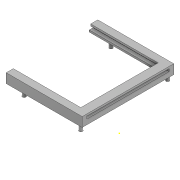
# Autodesk Inventor part: podstawa_2
Saved by Autodesk Inventor 2021 (Build 250183000, 183)
## iProperties
Created: 2022-06-23
Part Number: podstawa_2
Material: Generic
Document SubType Name: Modeling
Designer: agnpi
Density: 1 g/cm^3
Appearance: Orange
Author: agnpi
Autodesk Inventor part; units mm, degrees
ref_plane "YZ Plane" through (0, 0, 0) normal (1, 0, 0) x (0, 1, 0)
ref_plane "XZ Plane" through (0, 0, 0) normal (0, 1, 0) x (-1, 0, 0)
ref_plane "XY Plane" through (0, 0, 0) normal (0, 0, 1) x (1, 0, 0)
sketch "Sketch1" plane through (0, 0, 0) normal (0, 1, 0) x (-1, 0, 0)
  line L0 (164.8, 0) -> (-148.8, 0) projected
  line L1 (0, -144.2) -> (0, 144.2) projected
  line L2 (-80, 95) -> (80, 95)
  line L3 (80, 95) -> (80, -95)
  line L4 (80, -95) -> (-80, -95)
  line L5 (-80, -95) -> (-80, 95)
  line L6 (-80, 95) -> (80, -95) construction
  line L7 (80, 95) -> (-80, -95) construction
  line L8 (-88, 103) -> (88, 103)
  line L9 (88, 103) -> (88, -103)
  line L10 (88, -103) -> (-88, -103)
  line L11 (-88, -103) -> (-88, 103)
  point P0 (0, 0)
  dimension "d0" = 160
  dimension "d1" = 190
  dimension "d2" = 8
  dimension "d3" = 8
  dimension "d4" = 8
  dimension "d5" = 8
  constraints: 20 end point, 3 parallel, 3 perpendicular, 2 horizontal, 2 midpoint
  measures "d0" distance of L3.end L4.end
  measures "d1" distance of L2.end L3.end
  measures "d2" distance between parallel lines of L2 L8
  measures "d3" distance between parallel lines of L10 L4
  measures "d4" distance between parallel lines of L11 L5
  measures "d5" distance between parallel lines of L9 L3
extrude "Extrusion1" add sketch "Sketch1" along normal blind 8 contours L3 L4 L1 L0 | L0 L1 L2 L3 | L1 L4 L5 L0 | L0 L5 L2 L1
extrude "Extrusion2" add sketch "Sketch1" along normal blind 80 contours L9 L10 L1 L4 L3 L0 | L0 L3 L2 L1 L8 L9 | L1 L2 L5 L0 L11 L8 | L10 L11 L0 L5 L4 L1
move faces "Move1" translate (-16, 0, 0) faces at (80, 32, -31.6667)
move faces "Move5" translate (-8, 0, 0) faces at (88, 53.3333, 34.3333)
move faces "Move6" translate (-8, 0, 0) faces at (80, 53.3333, 34.3333)
move faces "Move7" translate (0, 0, -8) faces at (-32, 56, 95)
move faces "Move8" translate (0, 0, -8) faces at (-34.6667, 26.6667, 103)
move faces "Move9" translate (0, 0, -8) faces at (-32, 56, 87)
move faces "Move10" translate (0, 0, -8) faces at (-34.6667, 26.6667, 95)
thicken "Thicken1" operation add thickness 3 both sides no extend neighbours yes toward (0, 0, 1) faces at (-34.6667, 26.6667, 87)
thicken "Thicken3" operation add thickness 3 both sides no extend neighbours yes toward (0, 0, -1) faces at (18.6667, 26.6667, -103)
sketch "Sketch5" plane through (0, 8, 0) normal (0, 1, 0) x (1, 0, 0)
  line L0 (-80, -79) -> (-80, 95) projected
  line L1 (-80, 95) -> (64, 95) projected
  line L2 (-80, 89.3431) -> (-74.3431, 95)
  line L3 (-80, 89.3431) -> (-80, 95)
  line L4 (58.3431, 95) -> (64, 89.3431)
  line L5 (64, 95) -> (64, -79) projected
  line L6 (-80, -73.3431) -> (-74.3431, -79)
  line L7 (64, -79) -> (-80, -79) projected
  line L8 (58.3431, -79) -> (64, -73.3431)
  point P0 (0, 0)
  dimension "d69" = 45
  dimension "d70" = 8
  dimension "d73" = 8
  dimension "d74" = 45
  dimension "d75" = 8
  dimension "d76" = 45
  dimension "d77" = 8
  dimension "d78" = 45
  constraints: 10 end point, 8 point on line, 1 collinear
  measures "d69" angle of L2 L0
  measures "d70" distance of L2.start L2.end
  measures "d73" distance of L4.start L4.end
  measures "d74" angle of L5 L4
  measures "d75" distance of L6.start L6.end
  measures "d76" angle of L7 L6
  measures "d77" distance of L8.start L8.end
  measures "d78" angle of L7 L8
thicken "Thicken4" operation add thickness 1 both sides no extend neighbours yes toward (1, 0, 0) faces at (-80, 56, -37)
thicken "Thicken5" operation add thickness 1 both sides no extend neighbours yes toward (-1, 0, 0) faces at (64, 56, 21)
sketch "Sketch6" plane through (0, 0, 0) normal (0, -1, 0) x (1, 0, 0)
  line L0 (72, 90) -> (72, -106) projected
  line L1 (72, -106) -> (-88, -106) projected
  line L2 (72, 90) -> (-88, 90)
  line L3 (-88, 90) -> (-88, -106)
  line L4 (-88, -106) -> (72, -106)
  line L5 (72, -106) -> (72, 90)
  point P0 (0, 0)
  constraints: 8 end point, 2 parallel, 1 horizontal, 1 perpendicular
extrude "Extrusion7" cut sketch "Sketch6" against normal blind 45
sketch "Sketch7" plane through (-79, 80, 79) normal (1, 0, 0) x (0, 0, -1)
  line L0 (0, -35) -> (0, 0) projected
  line L1 (174, -13.5) -> (174, -21.5)
  line L2 (174, -21.5) -> (0, -21.5)
  line L3 (0, -21.5) -> (0, -13.5)
  line L4 (174, -35) -> (174, 0) projected
  line L5 (0, 0) -> (174, 0) projected
  line L6 (0, -13.5) -> (174, -13.5)
  point P0 (79, -80)
  point P1 (174, -17.5)
  point P2 (0, -21.5)
  dimension "d91" = 8
  constraints: 8 end point, 2 midpoint, 2 point on line, 1 horizontal, 1 parallel
  measures "d91" distance between parallel lines of L2 L6
extrude "Extrusion8" add sketch "Sketch7" along normal up to surface (142 mm away) contours L0 L6 L1 L2
sketch "Sketch8" plane through (-79, 66.5, 79) normal (0, 1, 0) x (1, 0, 0)
  line L0 (8, 166) -> (134, 166)
  line L1 (134, 166) -> (134, 8)
  line L2 (134, 8) -> (8, 8)
  line L3 (8, 8) -> (8, 166)
  line L4 (0, 174) -> (142, 174) projected
  line L5 (0, 0) -> (0, 174) projected
  line L6 (142, 0) -> (0, 0) projected
  line L7 (142, 174) -> (142, 0) projected
  point P0 (79, 79)
  dimension "d95" = 8
  dimension "d96" = 8
  dimension "d97" = 8
  dimension "d98" = 8
  constraints: 8 end point, 2 parallel, 1 horizontal, 1 perpendicular
  measures "d95" distance between parallel lines of L4 L0
  measures "d96" distance between parallel lines of L3 L5
  measures "d97" distance between parallel lines of L6 L2
  measures "d98" distance between parallel lines of L1 L7
extrude "Extrusion9" cut sketch "Sketch8" against normal through all contours L0 L1 L2 L3
sketch "Sketch10" plane through (-79, 80, 79) normal (1, 0, 0) x (0, 0, -1)
  line L0 (0, 0) -> (174, 0) projected
  line L1 (0, 0) -> (174, 0)
  line L2 (174, 0) -> (174, -4)
  line L3 (174, -4) -> (0, -4)
  line L4 (0, -4) -> (0, 0)
  line L5 (174, -13.5) -> (174, 0) projected
  point P0 (79, -80)
  point P1 (174, -6.75)
  dimension "d101" = 4
  constraints: 8 end point, 2 parallel, 1 horizontal, 1 midpoint, 1 perpendicular, 1 point on line
  measures "d101" distance between parallel lines of L0 L3
extrude "Extrusion10" add sketch "Sketch10" along normal up to surface (142 mm away)
sketch "Sketch11" plane through (0, 80, 0) normal (0, 1, 0) x (1, 0, 0)
  line L0 (53, 90) -> (-69, 90)
  line L1 (-69, 90) -> (-69, -74)
  line L2 (-69, -74) -> (53, -74)
  line L3 (53, -74) -> (53, 90)
  line L4 (72, -90) -> (72, 106) projected
  line L5 (72, 106) -> (-88, 106) projected
  line L6 (-88, -90) -> (72, -90) projected
  line L7 (-88, 106) -> (-88, -90) projected
  point P0 (0, 0)
  dimension "d104" = 19
  dimension "d105" = 16
  dimension "d106" = 16
  dimension "d107" = 19
  constraints: 8 end point, 2 parallel, 1 horizontal, 1 perpendicular
  measures "d104" distance between parallel lines of L4 L3
  measures "d105" distance between parallel lines of L5 L0
  measures "d106" distance between parallel lines of L6 L2
  measures "d107" distance between parallel lines of L7 L1
extrude "Extrusion11" cut sketch "Sketch11" against normal blind 8 contours L3 L2 L1 L0
sketch "Sketch12" plane through (63, 66.5, -95) normal (-1, 0, 0) x (0, 0, 1)
  line L0 (0, 0) -> (0, 9.5) projected
  line L1 (0, 0) -> (174, 0) projected
  line L2 (0, 9.5) -> (174, 9.5)
  line L3 (174, 9.5) -> (174, 0)
  line L4 (174, 0) -> (0, 0)
  line L5 (0, 0) -> (0, 9.5)
  point P0 (95, -66.5)
  constraints: 8 end point, 2 parallel, 1 horizontal, 1 perpendicular
extrude "Extrusion12" cut sketch "Sketch12" against normal through all
sketch "Sketch13" plane through (0, 80, 0) normal (0, 1, 0) x (1, 0, 0)
  line L0 (-69, 90) -> (-69, -74) projected
  line L1 (-69, -74) -> (-88, -74)
  line L2 (-69, 90) -> (-88, 90)
  line L3 (-88, -74) -> (-88, 90)
  line L4 (-88, 106) -> (-88, -90) projected
  line L5 (-69, 90) -> (-69, -74)
  point P0 (0, 0)
  constraints: 8 end point, 3 collinear, 2 horizontal
extrude "Extrusion13" cut sketch "Sketch13" against normal through all
sketch "Sketch14" plane through (-88, 80, -90) normal (0, 0, 1) x (1, 0, 0)
  line L0 (9, -13.5) -> (19, -13.5) projected
  line L1 (0, -35) -> (0, 0) projected
  line L2 (9, -13.5) -> (0, -13.5)
  line L3 (0, -13.5) -> (0, -4)
  line L4 (0, -4) -> (9, -4)
  line L5 (9, -4) -> (9, -13.5)
  point P0 (88, -80)
  constraints: 8 end point, 2 parallel, 2 point on line, 1 horizontal, 1 perpendicular
extrude "Extrusion14" cut sketch "Sketch14" against normal up to surface (5 mm away)
sketch "Sketch15" plane through (-69, 58.5, -90) normal (-1, 0, 0) x (0, 0, 1)
  line L0 (0, 8) -> (0, 0) projected
  line L1 (161, 0) -> (3, 0) projected
  line L2 (0, 8) -> (3, 8)
  line L3 (3, 8) -> (3, 0)
  line L4 (3, 0) -> (0, 0)
  line L5 (0, 0) -> (0, 8)
  point P0 (90, -58.5)
  constraints: 8 end point, 2 parallel, 1 horizontal, 1 perpendicular
extrude "Extrusion15" add sketch "Sketch15" along normal up to surface (19 mm away)
sketch "Sketch16" plane through (-69, 58.5, 71) normal (-1, 0, 0) x (0, 0, 1)
  line L0 (0, 8) -> (3, 8)
  line L1 (3, 8) -> (3, 0)
  line L2 (3, 0) -> (0, 0)
  line L3 (0, 0) -> (0, 8)
  point P0 (-71, -58.5)
  constraints: 8 end point, 2 parallel, 1 horizontal, 1 perpendicular
extrude "Extrusion16" add sketch "Sketch16" along normal up to surface (19 mm away)
sketch "Sketch17" plane through (53, 80, 74) normal (0, 0, -1) x (-1, 0, 0)
  line L0 (132, -13.5) -> (132, -4) projected
  line L1 (132, -13.5) -> (141, -13.5) projected
  line L2 (132, -4) -> (141, -4)
  line L3 (141, -4) -> (141, -13.5)
  line L4 (141, -13.5) -> (132, -13.5)
  line L5 (132, -13.5) -> (132, -4)
  line L6 (141, -35) -> (132, -35)
  line L7 (132, -35) -> (132, -21.5)
  line L8 (132, -21.5) -> (141, -21.5)
  line L9 (141, -21.5) -> (141, -35)
  line L10 (141, -21.5) -> (132, -21.5) projected
  point P0 (53, -80)
  point P1 (136.5, -21.5)
  dimension "d120" = 9
  constraints: 16 end point, 4 parallel, 2 horizontal, 2 midpoint, 2 perpendicular
  measures "d120" distance between parallel lines of L9 L7
extrude "Extrusion17" cut sketch "Sketch17" against normal up to surface (5 mm away)
move faces "Move11" translate (0, 0, 3) faces at (-34.6667, 56.6667, 90)
move faces "Move12" translate (0, 0, -3) faces at (18.6667, 56.6667, -106)
move faces "Move13" translate (1, 0, 0) faces at (72, 52.1667, 21)
sketch "Sketch18" plane through (0, 45, 0) normal (0, -1, 0) x (1, 0, 0)
  line L0 (-79, -95) -> (63, -95) projected
  line L1 (58.343, -95) -> (63, -90.343)
  line L2 (63, -95) -> (63, 79) projected
  line L3 (63, 74.343) -> (58.343, 79)
  line L4 (-88, 79) -> (73, 79) projected
  point P0 (0, 0)
  dimension "d132" = 45
  dimension "d133" = 45
  dimension "d134" = 6.586
  dimension "d135" = 6.586
  constraints: 4 end point, 4 point on line
  measures "d132" angle of L0 L1
  measures "d133" angle of L4 L3
  measures "d134" distance of L3.start L3.end
  measures "d135" distance of L1.start L1.end
extrude "Extrusion18" add sketch "Sketch18" against normal up to surface (13.5 mm away)
sketch "Sketch19" plane through (0, 45, 0) normal (0, -1, 0) x (1, 0, 0)
  circle A0 centre (65, 84) radius 3.5
  circle A1 centre (65, -100) radius 3.5
  line L0 (73, 93) -> (73, -109) projected
  line L1 (73, -109) -> (-88, -109) projected
  line L2 (-88, 93) -> (73, 93) projected
  line L3 (-88, 79) -> (58.343, 79) projected
  line L4 (-79, -95) -> (58.343, -95) projected
  point P0 (0, 0)
  dimension "d138" = 7
  dimension "d139" = 7
  dimension "d140" = 8
  dimension "d143" = 8
  dimension "d156" = 5
  dimension "d157" = 5
  constraints: 2 centre point
  measures "d138" diameter of A0
  measures "d139" diameter of A1
  measures "d140" distance from line of L0 A1.centre
  measures "d143" distance from line of L0 A0.centre
  measures "d156" distance from line of L3 A0.centre
  measures "d157" distance from line of L4 A1.centre
extrude "Extrusion19" add sketch "Sketch19" along normal blind 15
sketch "Sketch20" plane through (-88, 58.5, -90) normal (0, 0, 1) x (1, 0, 0)
  line L0 (9, -13.5) -> (146.343, -13.5) projected
  line L1 (0, -13.5) -> (0, 0) projected
  line L2 (9, -13.5) -> (0, -13.5)
  line L3 (0, -13.5) -> (0, 0)
  line L4 (0, 0) -> (9, 0)
  line L5 (9, 0) -> (9, -13.5)
  point P0 (88, -58.5)
  constraints: 8 end point, 2 parallel, 1 horizontal, 1 perpendicular
extrude "Extrusion20" cut sketch "Sketch20" against normal up to surface (5 mm away)
sketch "Sketch21" plane through (0, 45, 0) normal (0, -1, 0) x (1, 0, 0)
  circle A0 centre (-55, 84) radius 3.5
  line L0 (-88, 79) -> (73, 79) projected
  line L1 (-88, 93) -> (73, 93) projected
  circle A1 centre (65, 84) radius 3.5 projected
  circle A2 centre (-55, -100) radius 3.5
  line L2 (-88, -95) -> (58.343, -95) projected
  circle A3 centre (65, -100) radius 3.5 projected
  point P0 (0, 0)
  dimension "d148" = 7
  dimension "d150" = 120
  dimension "d151" = 7
  dimension "d153" = 120
  dimension "d158" = 5
  dimension "d159" = 5
  constraints: 2 centre point
  measures "d148" diameter of A0
  measures "d150" distance of A1.centre A0.centre
  measures "d151" diameter of A2
  measures "d153" distance of A3.centre A2.centre
  measures "d158" distance from line of L0 A0.centre
  measures "d159" distance from line of L2 A2.centre
extrude "Extrusion21" add sketch "Sketch21" along normal blind 15 contours A0 | A2
move faces "Move14" translate (0, 0, -4) faces at (-34.3333, 56.6667, 93)
move faces "Move15" translate (0, 0, 4) faces at (19.3333, 56.6667, -109)
move faces "Move17" translate (2, 0, 0) faces at (53, 77.3333, 19.3333)
sketch "Sketch22" plane through (-88, 66.5, 71) normal (0, 1, 0) x (1, 0, 0)
  line L0 (0, 158) -> (143, 158) projected
  line L1 (0, 166) -> (0, 158)
  line L2 (0, 158) -> (143, 158)
  line L3 (143, 158) -> (143, 0) projected
  line L4 (143, 158) -> (143, 0)
  line L5 (0, 0) -> (0, -8) projected
  line L6 (143, 0) -> (0, 0)
  line L7 (0, -8) -> (161, -8) projected
  line L8 (0, 0) -> (0, -8)
  line L9 (0, -8) -> (161, -8)
  line L10 (161, -8) -> (161, 166)
  line L11 (161, 166) -> (0, 166)
  line L12 (0, 166) -> (0, 158) projected
  line L13 (0, 166) -> (0, 158)
  point P0 (88, 71)
  constraints: 18 end point, 6 perpendicular, 3 collinear
extrude "Extrusion22" add sketch "Sketch22" along normal blind 4
move faces "Move20" translate (0, 8, 0) faces at (60.3333, 58.5, -34.3333)
move faces "Move21" translate (0, 15, 0) faces at (69.6667, 45, -35.4477)
move faces "Move22" translate (0, 15, 0) faces at (64.2375, 30, 82.2185)
move faces "Move23" translate (0, 15, 0) faces at (-55.8733, 30, 84.7736)
move faces "Move24" translate (0, 15, 0) faces at (-55.8733, 30, -99.2264)
move faces "Move25" translate (0, 15, 0) faces at (64.2375, 30, -101.7815)
move faces "Move26" translate (0, 3, 0) faces at (64.2375, 45, 82.2185) (-55.8733, 45, 84.7736)
move faces "Move27" translate (0, 3, 0) faces at (-55.8733, 48, 84.7736)
move faces "Move28" translate (0, 3, 0) faces at (-55.8733, 45, -99.2264)
move faces "Move29" translate (0, 3, 0) faces at (64.2375, 45, -101.7815)
body "Solid1"
